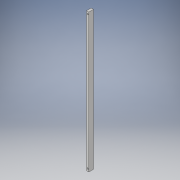
# Autodesk Inventor part: GlyphPlateRightSide
Saved by Autodesk Inventor 2017 (Build 210142000, 142)
## iProperties
Created: 2018-01-27
Part Number: GlyphPlateRightSide
Material: Generic
Document SubType Name: Modeling
Designer: User
Density: 1 g/cm^3
Appearance: Default
Author: User
Autodesk Inventor part; units mm, degrees
ref_plane "YZ Plane" through (0, 0, 0) normal (1, 0, 0) x (0, 1, 0)
ref_plane "XZ Plane" through (0, 0, 0) normal (0, 1, 0) x (-1, 0, 0)
ref_plane "XY Plane" through (0, 0, 0) normal (0, 0, 1) x (1, 0, 0)
sketch "Sketch1" plane through (0, 0, 0) normal (0, 0, 1) x (1, 0, 0)
  line L0 (0, 0) -> (6.35, 0)
  line L1 (6.35, 0) -> (6.35, 374.65)
  line L2 (6.35, 374.65) -> (0, 374.65)
  line L3 (0, 374.65) -> (0, 0)
  dimension "d0" = 6.35
  dimension "d1" = 374.65
  constraints: 8 end point, 2 parallel, 1 horizontal, 1 perpendicular
  measures "d0" distance of L2.end L1.end
  measures "d1" distance of L1.end L0.end
extrude "Extrusion1" add sketch "Sketch1" along normal blind 12.7
sketch "Sketch2" plane through (0, 0, 12.7) normal (0, 0, 1) x (1, 0, 0)
  line L0 (0, 0) -> (6.35, 0) projected
  line L1 (3.175, 0) -> (3.175, 6.35)
  circle A0 centre (3.175, 6.35) radius 1.778
  line L2 (6.35, 374.65) -> (0, 374.65) projected
  line L3 (3.175, 374.65) -> (3.175, 368.3)
  circle A1 centre (3.175, 368.3) radius 1.778
  dimension "d4" = 6.35
  dimension "d5" = 3.556
  dimension "d6" = 6.35
  dimension "d7" = 3.556
  constraints: 4 end point, 2 centre point, 2 coincident, 2 midpoint, 2 vertical
  measures "d4" distance of L1.start L1.end
  measures "d5" diameter of A0
  measures "d6" distance of L3.start L3.end
  measures "d7" diameter of A1
extrude "Extrusion2" cut sketch "Sketch2" against normal blind 12.7
body "Solid1"
